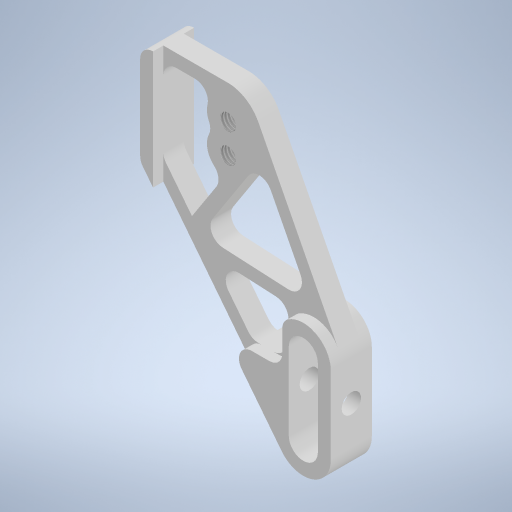
# Autodesk Inventor part: VerticalSlideMiddleBottom2.2
Saved by Autodesk Inventor 2023 (Build 270158000, 158)
## iProperties
Created: 2022-10-14
Part Number: VerticalSlideMiddleBottom2.2
Material: Generic
Document SubType Name: Modeling
Designer: deli
Density: 1 g/cm^3
Appearance: Default
Mass: 1.85178 g
Surface Area: 22.5906 cm^2
Volume: 1.85178 cm^3
Author: deli
Autodesk Inventor part; units mm, degrees
ref_plane "YZ Plane" through (0, 0, 0) normal (1, 0, 0) x (0, 1, 0)
ref_plane "XZ Plane" through (0, 0, 0) normal (0, 1, 0) x (-1, 0, 0)
ref_plane "XY Plane" through (0, 0, 0) normal (0, 0, 1) x (1, 0, 0)
sketch "Sketch1" plane through (0, 0, 0) normal (0, 0, 1) x (1, 0, 0)
  line L0 (-75.1619, -151.2747) -> (-75.1619, -164.2747)
  line L1 (-74.7357, -165.5089) -> (-53.2562, -192.8974)
  circle A0 centre (-63.1619, -159.0247) radius 1.25
  circle A1 centre (-63.1619, -154.5247) radius 1.25
  arc A2 (-52.1619, -190.2747) -> (-47.6619, -190.2747) centre (-49.9119, -190.2747) ccw
  arc A3 (-47.6619, -178.2747) -> (-52.1619, -178.2747) centre (-49.9119, -178.2747) ccw
  line L2 (-47.6619, -178.2747) -> (-47.6619, -190.2747)
  line L3 (-52.1619, -178.2747) -> (-52.1619, -190.2747)
  line L4 (-45.6619, -178.2747) -> (-45.6619, -190.2747)
  arc A4 (-53.2562, -192.8974) -> (-45.6619, -190.2747) centre (-49.9119, -190.2747) ccw
  arc A5 (-45.6619, -178.2747) -> (-46.1268, -176.3419) centre (-49.9119, -178.2747) ccw
  line L5 (-46.1268, -176.3419) -> (-58.4862, -152.1372)
  line L6 (-73.1619, -149.2747) -> (-63.1619, -149.2747)
  arc A6 (-58.4862, -152.1372) -> (-63.1619, -149.2747) centre (-63.1619, -154.5247) ccw
  arc A7 (-73.1619, -149.2747) -> (-75.1619, -151.2747) centre (-73.1619, -151.2747) ccw
  arc A8 (-75.1619, -164.2747) -> (-74.7357, -165.5089) centre (-73.1619, -164.2747) ccw
  line L7 (-52.1619, -182.7747) -> (-56.1619, -182.7747)
  line L8 (-56.1619, -182.7747) -> (-56.1619, -185.7747)
  line L9 (-56.1619, -185.7747) -> (-52.1619, -185.7747)
  point P0 (0, 0)
  dimension "d2" = 2.5
  dimension "d11" = 2
  dimension "d22" = 12
  dimension "d46" = 2
  dimension "d47" = 4.5
  dimension "d84" = 4
  dimension "d86" = 12
  dimension "d87" = 12
  dimension "d88" = 23
  dimension "d90" = 4
  dimension "d91" = 3
  dimension "d92" = 4.5
  dimension "d94" = 15
  dimension "d95" = 19.25
  dimension "d96" = 2
  constraints: 20 end point, 16 point on circle, 13 tangent, 9 centre point, 4 equal radius, 4 point on line, 3 perpendicular, 2 coincident, 2 vertical, 1 concentric, 1 horizontal, 1 parallel
  measures "d2" diameter of A0
  measures "d22" distance of A2.centre A3.centre
  measures "d46" radial gap between concentric circles of A4 A2
  measures "d47" distance between parallel lines of L2 L3
  measures "d84" distance edge to line of A1 L6
  measures "d86" distance from line of A1.centre L0
  measures "d87" distance from line of A0.centre L0
  measures "d88" distance between parallel lines of L3 L0
  measures "d90" distance of L7.start L7.end
  measures "d91" distance of L7.end L8.end
  measures "d92" distance from line of L3.start L7
  measures "d94" distance from line of L6 L0.end
  measures "d95" vertical distance of A3.centre A0.centre
  measures "d96" radius of A7
extrude "Extrusion1" add sketch "Sketch1" along normal blind 6.35 contours A7 L6 A6 L5 A5 L4 A4 L1 A8 L0 | L9 L8 L7 L3
thread "Thread2" size "M3x0.5" class "6H" standard "ANSI Metric M Profile" full length
thread "Thread6" size "M3x0.5" class "6H" standard "ANSI Metric M Profile" full length
sketch "Sketch8" plane through (-52.1619, -190.2747, 0) normal (1, 0, 0) x (0, 0, -1)
  line L0 (0, 0) -> (0, 12) construction
  line L1 (0, 12) -> (-6.35, 12) construction
  line L2 (-6.35, 0) -> (-6.35, 12) construction
  line L3 (0, 0) -> (-6.35, 0) construction
  line L4 (0, 0) -> (-6.35, 0) construction
  line L5 (-6.35, 12) -> (0, 0) construction
  line L6 (-6.35, 0) -> (0, 12) construction
  circle A0 centre (-3.175, 6) radius 1.5
  point P0 (0, 190.2747)
  dimension "d97" = 3
  constraints: 4 end point, 1 centre point, 1 midpoint
  measures "d97" diameter of A0
extrude "Extrusion7" cut sketch "Sketch8" along normal blind 10 and the other way blind 4
sketch "Sketch12" plane through (0, 0, 6.35) normal (0, 0, 1) x (1, 0, 0)
  line L0 (-75.1619, -151.2747) -> (-75.1619, -164.2747) projected
  arc A0 (-75.1619, -164.2747) -> (-74.7357, -165.5089) centre (-73.1619, -164.2747) ccw projected
  line L1 (-74.7357, -165.5089) -> (-53.2562, -192.8974) projected
  arc A1 (-53.2562, -192.8974) -> (-45.6619, -190.2747) centre (-49.9119, -190.2747) ccw projected
  line L2 (-45.6619, -190.2747) -> (-45.6619, -178.2747) projected
  arc A2 (-45.6619, -178.2747) -> (-46.1268, -176.3419) centre (-49.9119, -178.2747) ccw projected
  line L3 (-46.1268, -176.3419) -> (-58.4862, -152.1372) projected
  arc A3 (-58.4862, -152.1372) -> (-63.1619, -149.2747) centre (-63.1619, -154.5247) ccw projected
  line L4 (-63.1619, -149.2747) -> (-73.1619, -149.2747) projected
  arc A4 (-73.1619, -149.2747) -> (-75.1619, -151.2747) centre (-73.1619, -151.2747) ccw projected
  circle A5 centre (-63.1619, -159.0247) radius 1.25 projected
  circle A6 centre (-63.1619, -154.5247) radius 1.25 projected
  line L5 (-47.6619, -178.2747) -> (-47.6619, -190.2747) projected
  arc A7 (-52.1619, -190.2747) -> (-47.6619, -190.2747) centre (-49.9119, -190.2747) ccw projected
  line L6 (-52.1619, -190.2747) -> (-52.1619, -178.2747) projected
  arc A8 (-47.6619, -178.2747) -> (-52.1619, -178.2747) centre (-49.9119, -178.2747) ccw projected
  line L7 (-60.2675, -153.0467) -> (-49.5477, -174.0403)
  line L8 (-54.1619, -188.5015) -> (-73.1619, -164.2747)
  line L9 (-73.1619, -164.2747) -> (-73.1619, -151.2747)
  line L10 (-73.1619, -151.2747) -> (-63.1619, -151.2747)
  arc A9 (-65.5072, -156.7747) -> (-60.8167, -156.7747) centre (-63.1619, -159.0247) ccw
  line L11 (-54.1619, -178.2747) -> (-54.1619, -188.5015)
  arc A10 (-63.1619, -151.2747) -> (-65.5072, -156.7747) centre (-63.1619, -154.5247) ccw
  arc A11 (-60.8167, -156.7747) -> (-60.2675, -153.0467) centre (-63.1619, -154.5247) ccw
  arc A12 (-49.5477, -174.0403) -> (-54.1619, -178.2747) centre (-49.9119, -178.2747) ccw
  line L12 (-52.1619, -181.7747) -> (-59.9467, -181.7747)
  line L13 (-67.4296, -171.584) -> (-58.1289, -157.2349)
  line L14 (-67.4296, -171.584) -> (-50.3526, -172.4641)
  line L15 (-63.7448, -162.222) -> (-68.7345, -169.9201)
  line L16 (-65.7928, -173.671) -> (-51.6572, -174.3995)
  point P0 (0, 0)
  point P1 (-72.1199, -165.6034)
  point P2 (-55.0939, -163.1786)
  point P3 (-61.507, -179.1359)
  point P4 (-60.0818, -180.9531)
  point P5 (-53.8878, -165.5408)
  point P6 (-73.1619, -163.7316)
  point P7 (-59.4375, -181.7747)
  point P8 (-54.1619, -181.7747)
  dimension "d108" = 2
  dimension "d110" = 2
  dimension "d111" = 2
  dimension "d112" = 2
  dimension "d113" = 2
  dimension "d114" = 2
  dimension "d115" = 2
  dimension "d116" = 2
  dimension "d124" = 3.5
  dimension "d132" = 60
  dimension "d133" = 60
  dimension "d134" = 2
  dimension "d135" = 2
  constraints: 21 end point, 12 point on line, 10 point on circle, 4 centre point, 2 parallel, 1 horizontal, 1 tangent, 1 other
  measures "d108" distance between parallel lines of L3 L7
  measures "d110" radial gap between concentric circles of A5 A9
  measures "d111" distance between parallel lines of L6 L11
  measures "d112" radial gap between concentric circles of A6 A10
  measures "d113" radial gap between concentric circles of A6 A11
  measures "d114" radial gap between concentric circles of A8 A12
  measures "d115" distance between parallel lines of L1 L8
  measures "d116" distance between parallel lines of L0 L9
  measures "d124" distance from line of A2.centre L12
  measures "d132" angle of L14 L13
  measures "d133" angle of L7 L14
  measures "d134" distance between parallel lines of L13 L15
  measures "d135" distance between parallel lines of L14 L16
extrude "Extrusion10" cut sketch "Sketch12" against normal blind 10 contours L7 L14 L13 | L15 L8 L9 L10 A10 A9 | A12 L11 L12 L8 L16
fillet "Fillet6" radius 2 12 edges at (-73.1619, -151.2747, 3.175) (-63.1619, -151.2747, 3.175) (-65.5072, -156.7747, 3.175) (-59.4375, -181.7747, 3.175) (-54.1619, -181.7747, 3.175) (-73.1619, -164.2747, 3.175) (-63.7448, -162.222, 3.175) (-50.3526, -172.4641, 3.175) (-67.4296, -171.584, 3.175) (-58.1289, -157.2349, 3.175) (-51.6572, -174.3995, 3.175) (-65.7928, -173.671, 3.175)
sketch "Sketch13" plane through (0, 0, 6.35) normal (0, 0, 1) x (1, 0, 0)
  line L0 (-73.1619, -146.4996) -> (-53.1619, -146.4996)
  line L1 (-53.1619, -146.4996) -> (-53.1619, -181.7747)
  line L2 (-53.1619, -181.7747) -> (-73.1619, -181.7747)
  line L3 (-73.1619, -181.7747) -> (-73.1619, -146.4996)
  line L4 (-75.1619, -151.2747) -> (-75.1619, -164.2747) projected
  line L5 (-52.1619, -190.2747) -> (-52.1619, -178.2747) projected
  line L6 (-56.1619, -181.7747) -> (-58.4643, -181.7747) projected
  arc A0 (-47.6619, -178.2747) -> (-52.1619, -178.2747) centre (-49.9119, -178.2747) ccw projected
  arc A1 (-45.6619, -178.2747) -> (-54.1619, -178.2747) centre (-49.9119, -178.2747) ccw
  line L7 (-54.1619, -178.2747) -> (-54.1619, -190.2747)
  line L8 (-46.1268, -176.3419) -> (-58.4862, -152.1372) projected
  point P0 (0, 0)
  point P1 (-53.1619, -175.5361)
  point P2 (-53.1619, -162.5643)
  dimension "d125" = 2
  dimension "d126" = 1
  constraints: 10 end point, 2 parallel, 2 point on circle, 1 centre point, 1 collinear, 1 horizontal, 1 perpendicular, 1 tangent, 1 other
  measures "d125" distance between parallel lines of L4 L3
  measures "d126" distance between parallel lines of L5 L1
extrude "Extrusion11" cut sketch "Sketch13" against normal blind 1.5875
sketch "Sketch14" plane through (0, 0, 0) normal (0, 0, -1) x (-1, 0, 0)
  circle A0 centre (63.1619, -159.0247) radius 1.25 projected
  circle A1 centre (63.1619, -154.5247) radius 1.25 projected
  line L0 (72.7357, -164.8182) -> (68.7345, -169.9201) projected
  arc A2 (53.1619, -175.5361) -> (46.1268, -176.3419) centre (49.9119, -178.2747) ccw projected
  line L1 (58.4862, -152.1372) -> (46.1268, -176.3419) projected
  arc A3 (63.1619, -149.2747) -> (58.4862, -152.1372) centre (63.1619, -154.5247) ccw projected
  line L2 (73.1619, -149.2747) -> (63.1619, -149.2747) projected
  line L3 (73.1619, -153.2747) -> (73.1619, -149.2747) projected
  arc A4 (73.1619, -153.2747) -> (71.1619, -151.2747) centre (71.1619, -153.2747) ccw projected
  line L4 (68.261, -151.2747) -> (71.1619, -151.2747) projected
  arc A5 (68.261, -151.2747) -> (66.3185, -153.7509) centre (68.261, -153.2747) ccw projected
  arc A6 (66.0983, -155.9175) -> (66.3185, -153.7509) centre (63.1619, -154.5247) ccw projected
  arc A7 (66.0983, -155.9175) -> (66.0983, -157.6318) centre (67.9054, -156.7747) ccw projected
  arc A8 (65.3011, -161.4714) -> (66.0983, -157.6318) centre (63.1619, -159.0247) ccw projected
  line L5 (73.1619, -167.5156) -> (73.1619, -163.5839) projected
  line L6 (61.9792, -181.7747) -> (73.1619, -167.5156) projected
  line L7 (58.4643, -181.7747) -> (61.9792, -181.7747) projected
  line L8 (51.9279, -169.3789) -> (56.5535, -160.3201) projected
  line L9 (54.1619, -179.7747) -> (54.1619, -178.2747) projected
  line L10 (53.1619, -181.7747) -> (56.1619, -181.7747) projected
  line L11 (53.1619, -175.5361) -> (53.1619, -181.7747) projected
  arc A9 (54.1619, -179.7747) -> (56.1619, -181.7747) centre (56.1619, -179.7747) ccw projected
  line L12 (55.7006, -174.1911) -> (61.4044, -173.8972) projected
  line L13 (68.7345, -169.9201) -> (64.9393, -164.0649) projected
  arc A10 (58.4643, -181.7747) -> (60.0381, -181.0089) centre (58.4643, -179.7747) ccw projected
  line L14 (63.0811, -177.1287) -> (60.0381, -181.0089) projected
  line L15 (63.9701, -171.7623) -> (53.8121, -172.2858) projected
  line L16 (60.013, -160.1418) -> (65.5454, -168.6771) projected
  arc A11 (65.3011, -161.4714) -> (64.9393, -164.0649) centre (66.6176, -162.977) ccw projected
  arc A12 (72.7357, -164.8182) -> (73.1619, -163.5839) centre (71.1619, -163.5839) ccw projected
  arc A13 (63.0811, -177.1287) -> (61.4044, -173.8972) centre (61.5073, -175.8945) ccw projected
  arc A14 (55.7006, -174.1911) -> (53.9182, -176.8561) centre (55.8035, -176.1885) ccw projected
  arc A15 (54.1619, -178.2747) -> (53.9182, -176.8561) centre (49.9119, -178.2747) ccw projected
  arc A16 (60.013, -160.1418) -> (56.5535, -160.3201) centre (58.3348, -161.2296) ccw projected
  arc A17 (51.9279, -169.3789) -> (53.8121, -172.2858) centre (53.7091, -170.2885) ccw projected
  arc A18 (63.9701, -171.7623) -> (65.5454, -168.6771) centre (63.8671, -169.7649) ccw projected
  point P0 (0, 0)
extrude "Extrusion12" cut sketch "Sketch14" against normal blind 1.5875 contours A12 L5 L6 L7 A10 L14 A13 L12 A14 A15 L9 A9 L10 L11 A2 L1 A3 L2 L3 A4 L4 A5 A6 A7 A8 A11 L13 L0 | L8 A16 L16 A18 L15 A17
fillet "Fillet7" radius 2 4 edges at (-53.1619, -175.5361, 5.5562) (-61.9792, -181.7747, 5.5562) (-61.9792, -181.7747, 0.7937) (-53.1619, -181.7747, 5.5562)
equation "\"d22\" = d17"
equation "\"d17\" = 12"
body "Solid1"
